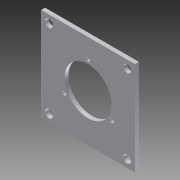
# Autodesk Inventor part: Top Plate BD Motor mount
Saved by Autodesk Inventor 2012 (Build 160160000, 160)
## iProperties
Created: 2012-06-30
Part Number: Top Plate BD Motor mount
Material: Default
Document SubType Name: Modeling
Designer: Bruce
Density: 1 g/cm^3
Author: Bruce
Autodesk Inventor part; units mm, degrees
ref_plane "YZ Plane" through (0, 0, 0) normal (1, 0, 0) x (0, 1, 0)
ref_plane "XZ Plane" through (0, 0, 0) normal (0, 1, 0) x (-1, 0, 0)
ref_plane "XY Plane" through (0, 0, 0) normal (0, 0, 1) x (1, 0, 0)
sketch "Sketch1" plane through (0, 0, 0) normal (0, 0, 1) x (1, 0, 0)
  line L0 (-38.1, 38.1) -> (38.1, 38.1)
  line L1 (38.1, 38.1) -> (38.1, -38.1)
  line L2 (38.1, -38.1) -> (-38.1, -38.1)
  line L3 (-38.1, -38.1) -> (-38.1, 38.1)
  circle A0 centre (0, 0) radius 19.05
  point P0 (-31.75, 31.75)
  point P1 (31.75, 31.75)
  point P2 (31.75, -31.75)
  point P3 (-31.75, -31.75)
  dimension "d0" = 76.2
  dimension "d1" = 76.2
  dimension "d2" = 38.1
  dimension "d3" = 38.1
  dimension "d4" = 38.1
  dimension "d5" = 6.35
  dimension "d6" = 6.35
  dimension "d7" = 6.35
  dimension "d8" = 6.35
  constraints: 8 end point, 2 horizontal alignment, 2 parallel, 2 vertical alignment, 1 centre point, 1 coincident, 1 horizontal, 1 perpendicular
  measures "d0" distance of L2.end L0.start
  measures "d1" distance of L1.end L2.end
  measures "d2" distance from line of L3 point (0, 0)
  measures "d3" distance from line of point (0, 0) L2
  measures "d4" diameter of A0
  measures "d5" distance from line of L0 point (-31.75, 31.75)
  measures "d6" distance from line of L3 point (-31.75, 31.75)
  measures "d7" distance from line of point (31.75, 31.75) L1
  measures "d8" distance from line of L2 point (-31.75, -31.75)
extrude "Extrusion1" add sketch "Sketch1" against normal blind 3.175
hole "Hole1" at (-31.75, 31.75, 0) at (31.75, 31.75, 0) at (31.75, -31.75, 0) at (-31.75, -31.75, 0) direction (0, 0, -1) diameter 6.35 end through all
sketch "Sketch2" plane through (0, 0, 0) normal (0, 0, 1) x (1, 0, 0)
  circle A0 centre (0, 0) radius 19.05 projected
  line L0 (-38.1, 38.1) -> (38.1, 38.1) projected
  line L1 (-38.1, -38.1) -> (-38.1, 38.1) projected
  line L2 (38.1, -38.1) -> (-38.1, -38.1) projected
  line L3 (38.1, 38.1) -> (38.1, -38.1) projected
  circle A1 centre (0, 0) radius 19.05 projected
  circle A2 centre (0, 0) radius 22.3343
  point P0 (0, 22.3343)
  point P1 (19.3421, -11.1672)
  point P2 (-19.3421, -11.1672)
  dimension "d19" = 38.6842
  dimension "d20" = 38.6842
  dimension "d21" = 38.6842
  dimension "d22" = 44.6687
  dimension "d24" = 38.1
  constraints: 3 point on circle, 1 centre point, 1 coincident
  measures "d19" distance of A2.end A2.start
  measures "d20" distance of point (-19.342, -11.167) A2.end
  measures "d21" distance of point (-19.342, -11.167) A2.start
  measures "d22" diameter of A2
  measures "d24" distance from line of L1 A2.start
hole "Hole2" at (0, 22.3343, 0) at (19.3421, -11.1672, 0) at (-19.3421, -11.1672, 0) direction (0, 0, -1) diameter 3.175 end through all
equation "\"d2\" = 0.5 * d1"
equation "\"d3\" = 0.5 * d0"
equation "\"d7\" = d6"
equation "\"d8\" = d5"
equation "\"d20\" = d19"
equation "\"d21\" = d19"
equation "\"d24\" = 0.5 * d1"
body "Solid1"
